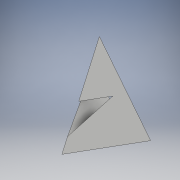
# Autodesk Inventor part: Задача №2
Saved by Autodesk Inventor 2019.1 (Build 231200000, 200)
## iProperties
Created: 2019-10-11
Part Number: Задача №2
Material: Типовые
Document SubType Name: Modeling
Designer: Stas
Density: 1 g/cm^3
Appearance: По умолчанию
Mass: 71.8384 g
Surface Area: 162.527 cm^2
Volume: 71.8384 cm^3
Author: Stas
Autodesk Inventor part; units mm, degrees
ref_plane "YZ Plane" through (0, 0, 0) normal (1, 0, 0) x (0, 1, 0)
ref_plane "XY Plane" through (0, 0, 0) normal (0, 0, 1) x (1, 0, 0)
sketch "Эскиз1" plane through (0, 0, 0) normal (0, 1, 0) x (-1, 0, 0)
  line L0 (0, 45) -> (38.9711, -22.5)
  line L1 (38.9711, -22.5) -> (-38.9711, -22.5)
  line L2 (-38.9711, -22.5) -> (0, 45)
  point P0 (0, 0)
  point P1 (0, 0)
  constraints: 6 end point, 1 coincident, 7 other
ref_plane "РабПлоскость2" through (0, 100, 0) normal (0, 1, 0) x (-1, 0, 0)
ref_plane "РабПлоскость1" through (0, 0, 0) normal (0, 1, 0) x (-1, 0, 0)
sketch "Эскиз2" plane through (0, 100, 0) normal (0, 1, 0) x (-1, 0, 0)
  point P0 (0, 0)
  point P1 (0, 0)
  constraints: 1 coincident
loft "Лофт1" add profiles "Эскиз1" section 2 point at (0, 100, 0)
sketch "Эскиз3" plane through (0, 0, 0) normal (0, 0, 1) x (1, 0, 0)
  point P0 (0, 0)
sketch "Эскиз4" plane through (0, 0, 0) normal (0, 0, 1) x (1, 0, 0)
  line L0 (0, 45) -> (15, 45)
  line L1 (15, 45) -> (-15, 45)
  line L2 (-15, 45) -> (0, 15)
  line L3 (15, 45) -> (0, 15)
  point P0 (0, 0)
  constraints: 8 end point, 1 point on line
extrude "Выдавливание1" cut sketch "Эскиз4" along normal through all both and the other way through all
